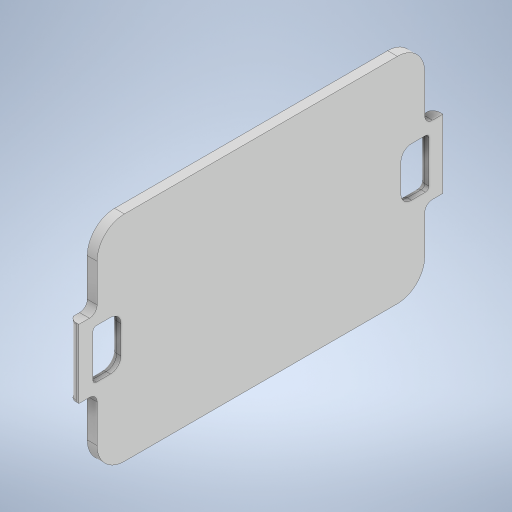
# Autodesk Inventor part: PlateGantryMountSpringRetainer
Saved by Autodesk Inventor 2023 (Build 270158000, 158)
## iProperties
Created: 2026-01-31
Part Number: PlateGantryMountSpringRetainer
Material: Generic
Document SubType Name: Modeling
Designer: DanAr
Density: 1 g/cm^3
Appearance: Default
Author: DanAr
Autodesk Inventor part; units mm, degrees
ref_plane "YZ Plane" through (0, 0, 0) normal (1, 0, 0) x (0, 1, 0)
ref_plane "XZ Plane" through (0, 0, 0) normal (0, 1, 0) x (-1, 0, 0)
ref_plane "XY Plane" through (0, 0, 0) normal (0, 0, 1) x (1, 0, 0)
sketch "Sketch1" plane through (0, 0, 0) normal (1, 0, 0) x (0, 1, 0)
  line L0 (-15.3, 23.4) -> (15.3, 23.4)
  line L1 (15.3, 23.4) -> (15.3, -23.4)
  line L2 (15.3, -23.4) -> (-15.3, -23.4)
  line L3 (-15.3, -23.4) -> (-15.3, 23.4)
  line L4 (-15.3, 23.4) -> (15.3, -23.4) construction
  line L5 (15.3, 23.4) -> (-15.3, -23.4) construction
  line L6 (-4.9, -26) -> (4.9, -26)
  line L7 (4.9, -26) -> (4.9, 26)
  line L8 (4.9, 26) -> (-4.9, 26)
  line L9 (-4.9, 26) -> (-4.9, -26)
  line L10 (-4.9, -26) -> (4.9, 26) construction
  line L11 (4.9, -26) -> (-4.9, 26) construction
  point P0 (0, 0)
  point P1 (-4.9, -23.4)
  point P2 (4.9, -23.4)
  point P3 (4.9, 23.4)
  point P4 (-4.9, 23.4)
  dimension "d0" = 46.8
  dimension "d1" = 30.6
  dimension "d2" = 52
  dimension "d3" = 9.8
  constraints: 24 end point, 4 midpoint, 4 parallel, 2 horizontal, 2 perpendicular
  measures "d0" distance of L0.end L1.end
  measures "d1" distance of L0.start L0.end
  measures "d2" distance of L6.end L7.end
  measures "d3" distance of L7.end L8.end
extrude "Extrusion1" add sketch "Sketch1" along normal blind 1.4
fillet "Fillet1" radius 1.1 4 edges at (0.7, 4.9, 23.4) (0.7, -4.9, 23.4) (0.7, 4.9, -23.4) (0.7, -4.9, -23.4)
fillet "Fillet2" radius 3.9 4 edges at (0.7, 15.3, 23.4) (0.7, 15.3, -23.4) (0.7, -15.3, 23.4) (0.7, -15.3, -23.4)
sketch "Sketch2" plane through (1.4, 0, 0) normal (1, 0, 0) x (0, 0, -1)
  line L0 (-26, 4.9) -> (-26, -4.9) projected
  line L1 (-26, 0) -> (-24, 0)
  line L2 (-24, 0) -> (-22, 0)
  line L3 (-20, -3.5) -> (-24, -3.5)
  line L4 (-24, -3.5) -> (-24, 3.5)
  line L5 (-24, 3.5) -> (-20, 3.5)
  line L6 (-20, 3.5) -> (-20, -3.5)
  line L7 (-20, -3.5) -> (-24, 3.5) construction
  line L8 (-24, -3.5) -> (-20, 3.5) construction
  line L9 (26, -4.9) -> (26, 4.9) projected
  line L10 (26, 0) -> (24, 0)
  line L11 (24, 0) -> (22, 0)
  line L12 (20, -3.5) -> (24, -3.5)
  line L13 (24, -3.5) -> (24, 3.5)
  line L14 (24, 3.5) -> (20, 3.5)
  line L15 (20, 3.5) -> (20, -3.5)
  line L16 (20, -3.5) -> (24, 3.5) construction
  line L17 (24, -3.5) -> (20, 3.5) construction
  point P0 (0, 0)
  dimension "d8" = 2
  dimension "d9" = 2
  dimension "d10" = 4
  dimension "d11" = 7
  dimension "d12" = 2
  dimension "d13" = 2
  dimension "d14" = 4
  dimension "d15" = 7
  constraints: 32 end point, 6 midpoint, 5 horizontal, 4 parallel, 2 perpendicular, 1 point on line
  measures "d8" distance of L1.start L1.end
  measures "d9" distance of L1.end L2.end
  measures "d10" distance of L4.end L5.end
  measures "d11" distance of L3.end L4.end
  measures "d12" distance of L10.start L10.end
  measures "d13" distance of L10.end L11.end
  measures "d14" distance of L13.end L14.end
  measures "d15" distance of L12.end L13.end
extrude "Extrusion2" cut sketch "Sketch2" against normal blind 1.4
fillet "Fillet3" radius 0.5 4 edges at (0.7, -3.5, -24) (0.7, 3.5, -24) (0.7, 3.5, 24) (0.7, -3.5, 24)
fillet "Fillet4" radius 1.5 4 edges at (0.7, -3.5, 20) (0.7, 3.5, 20) (0.7, 3.5, -20) (0.7, -3.5, -20)
fillet "Fillet5" radius 0.8 16 edges at (0, 0, 20) (0, 3.0607, 20.4393) (0, 3.5, 22.5) (0, 3.3536, 23.8536) (0, 0, 24) (0, -3.3536, 23.8536) (0, -3.5, 22.5) (0, -3.0607, 20.4393) (0, 3.3536, -23.8536) (0, 3.5, -22.5) (0, 3.0607, -20.4393) (0, 0, -20) (0, -3.0607, -20.4393) (0, -3.5, -22.5) (0, -3.3536, -23.8536) (0, 0, -24)
sketch "Sketch3" plane through (0, -4.9, 26) normal (0, 0, 1) x (1, 0, 0)
  line L0 (9.5754, -0.1) -> (-9.5754, -0.1)
  line L1 (-9.5754, -0.1) -> (-9.5754, 9.9)
  line L2 (-9.5754, 9.9) -> (9.5754, 9.9)
  line L3 (9.5754, 9.9) -> (9.5754, -0.1)
  line L4 (9.5754, -0.1) -> (-9.5754, 9.9) construction
  line L5 (-9.5754, -0.1) -> (9.5754, 9.9) construction
  line L6 (0, 10.9) -> (1.4, 10.9) projected
  line L7 (-19.1508, -1.1) -> (0, -1.1)
  line L8 (0, -1.1) -> (0, 10.9)
  line L9 (0, 10.9) -> (-19.1508, 10.9)
  line L10 (-19.1508, 10.9) -> (-19.1508, -1.1)
  line L11 (-19.1508, -1.1) -> (0, 10.9) construction
  line L12 (0, -1.1) -> (-19.1508, 10.9) construction
  line L13 (0, -1.1) -> (1.4, -1.1) projected
  line L14 (0, 10.9) -> (1.4, 10.9)
  line L15 (1.4, 10.9) -> (1.4, -1.1)
  line L16 (1.4, -1.1) -> (0, -1.1)
  line L17 (0, -1.1) -> (0, 10.9)
  line L18 (1.4, 9.8) -> (0, 9.8) projected
  line L19 (1.4, 0) -> (1.4, 9.8) projected
  line L20 (0, 9.8) -> (1.4, 9.8)
  line L21 (1.4, 9.8) -> (1.4, 0)
  line L22 (1.4, 0) -> (0, 0)
  line L23 (0, 0) -> (0, 9.8)
  line L24 (0, -3.3408) -> (-19.1508, -3.3408)
  line L25 (-19.1508, -3.3408) -> (-19.1508, 13.1408)
  line L26 (-19.1508, 13.1408) -> (0, 13.1408)
  line L27 (0, 13.1408) -> (0, -3.3408)
  line L28 (0, -3.3408) -> (-19.1508, 13.1408) construction
  line L29 (-19.1508, -3.3408) -> (0, 13.1408) construction
  line L30 (1.4, -6.5) -> (1.4, -1.1) projected
  line L31 (0, 13.1408) -> (1.4, 13.1408)
  line L32 (1.4, 13.1408) -> (1.4, -3.3408)
  line L33 (1.4, -3.3408) -> (0, -3.3408)
  line L34 (0, -3.3408) -> (0, 13.1408)
  point P0 (0, 4.9)
  point P1 (-9.5754, 4.9)
  point P2 (0, -0.1)
  point P3 (0, 9.9)
  point P4 (0, -3.3408)
  dimension "d21" = 10
  dimension "d29" = 12
  constraints: 60 end point, 12 parallel, 7 midpoint, 6 horizontal, 6 perpendicular, 1 point on line
  measures "d21" distance of L0.end L1.end
  measures "d29" distance of L9.end L7.start
extrude "Extrusion3" add sketch "Sketch3" against normal blind 2.5 contours L15 L13 L8 L0 | L0 L8 L22 L15 | L8 L7 L10 L9 L2 L1 L0 | L30 L33 L27 L13 | L15 L18 L8 L2 | L2 L8 L6 L15 | L27 L24 L25 L7 | L6 L27 L31 L32 | L9 L25 L26 L27
sketch "Sketch4" plane through (0, -4.9, -26) normal (0, 0, -1) x (-1, 0, 0)
  line L0 (9.5754, 9.9) -> (0, 9.9) projected
  line L1 (0, -0.1) -> (9.5754, -0.1) projected
  line L2 (9.5754, 9.9) -> (0, 9.9)
  line L3 (0, 9.9) -> (0, -0.1)
  line L4 (0, -0.1) -> (9.5754, -0.1)
  line L5 (9.5754, -0.1) -> (9.5754, 9.9)
  line L6 (0, 0) -> (-1.4, 0) projected
  line L7 (0, -0.1) -> (-1.4, -0.1)
  line L8 (-1.4, -0.1) -> (-1.4, 0)
  line L9 (-1.4, 0) -> (0, 0)
  line L10 (0, 0) -> (0, -0.1)
  line L11 (-1.4, -0.1) -> (9.5754, -0.1)
  line L12 (9.5754, -0.1) -> (9.5754, -1.1)
  line L13 (9.5754, -1.1) -> (-1.4, -1.1)
  line L14 (-1.4, -1.1) -> (-1.4, -0.1)
  line L15 (0, 9.9) -> (0, -0.1) projected
  line L16 (-1.4, 9.8) -> (0, 9.8) projected
  line L17 (0, 9.9) -> (-1.4, 9.9)
  line L18 (-1.4, 9.9) -> (-1.4, 9.8)
  line L19 (-1.4, 9.8) -> (0, 9.8)
  line L20 (0, 9.8) -> (0, 9.9)
  line L21 (-1.4, 10.9) -> (19.1508, 10.9) projected
  line L22 (-1.4, 9.9) -> (9.5754, 9.9)
  line L23 (9.5754, 9.9) -> (9.5754, 10.9)
  line L24 (9.5754, 10.9) -> (-1.4, 10.9)
  line L25 (-1.4, 10.9) -> (-1.4, 9.9)
  line L26 (19.1508, 10.9) -> (-1.4, 10.9) projected
  line L27 (-1.4, 10.9) -> (9.5754, 10.9)
  line L28 (9.5754, 10.9) -> (9.5754, 11.6514)
  line L29 (9.5754, 11.6514) -> (-1.4, 11.6514)
  line L30 (-1.4, 11.6514) -> (-1.4, 10.9)
  line L31 (-1.4, -1.1) -> (0, -1.1) projected
  line L32 (-1.4, -1.1) -> (9.5754, -1.1)
  line L33 (9.5754, -1.1) -> (9.5754, -1.8821)
  line L34 (9.5754, -1.8821) -> (-1.4, -1.8821)
  line L35 (-1.4, -1.8821) -> (-1.4, -1.1)
  point P0 (0, 4.9)
  constraints: 56 end point, 14 parallel, 7 horizontal, 7 perpendicular, 4 point on line
extrude "Extrusion4" add sketch "Sketch4" against normal blind 2.5 contours L0 L17 L25 L21 L23 | L3 L16 L18 L17 | L12 L13 L14 L7 L1 | L21 L30 L29 L28 | L7 L8 L6 L3 | L33 L34 L35 L13
fillet "Fillet7" radius 0.3 4 edges at (0, -5, -24.75) (0, 5, -24.75) (0, -5, 24.75) (0, 5, 24.75)
fillet "Fillet8" radius 1 9 edges at (-4.9377, -5, -26) (-0.0879, -4.9121, -26) (0, 0, -26) (-0.0879, 4.9121, -26) (-4.9377, 5, -26) (-0.0879, -4.9121, -23.5) (-4.9377, -5, -23.5) (-0.0879, 4.9121, -23.5) (-4.9377, 5, -23.5)
fillet "Fillet9" radius 1 9 edges at (-4.9377, -5, 23.5) (-0.0879, -4.9121, 23.5) (-0.0879, -4.9121, 26) (0, 0, 26) (-0.0879, 4.9121, 26) (-4.9377, 5, 26) (-4.9377, -5, 26) (-0.0879, 4.9121, 23.5) (-4.9377, 5, 23.5)
sketch "Sketch5" plane through (0, 0, 0) normal (-1, 0, 0) x (0, 0, 1)
  arc A0 (-23.5, 5.5417) -> (-23.4, 6) centre (-24.5, 6) ccw projected
  circle A1 centre (-24.5, 6) radius 1.1
  line L0 (-26, 6.7514) -> (-23.5, 6.7514) projected
  arc A2 (-24.5, 5) -> (-23.5, 6) centre (-24.5, 6) ccw projected
  line L1 (-26, 6.7514) -> (-23.5, 6.7514)
  line L2 (-23.5, 6.7514) -> (-23.5, 6)
  line L3 (-23.5, 6) -> (-26, 6)
  line L4 (-26, 6) -> (-26, 6.7514)
  line L5 (-24.5, 5) -> (-24.5, 4.7) projected
  line L6 (-26, 6.7514) -> (-26, -6.7821) projected
  line L7 (-24.5, 4.9) -> (-26, 4.9)
  line L8 (-26, 4.9) -> (-26, 6.7514)
  line L9 (-26, 6.7514) -> (-24.5, 6.7514)
  line L10 (-24.5, 6.7514) -> (-24.5, 4.9)
  arc A3 (-23.4, -6) -> (-23.977, -5.0323) centre (-24.5, -6) ccw projected
  circle A4 centre (-24.5, -6) radius 1.1
  line L11 (-24.5, -4.7) -> (-24.5, -5) projected
  line L12 (-24.5, -4.9) -> (-26, -4.9)
  line L13 (-26, -4.9) -> (-26, -6.7821)
  line L14 (-26, -6.7821) -> (-24.5, -6.7821)
  line L15 (-24.5, -6.7821) -> (-24.5, -4.9)
  line L16 (-23.5, -6.7821) -> (-26, -6.7821)
  line L17 (-26, -6.7821) -> (-26, -4.9)
  line L18 (-26, -4.9) -> (-23.5, -4.9)
  line L19 (-23.5, -4.9) -> (-23.5, -6.7821)
  point P0 (0, 0)
  point P1 (-23.5, 6.4583)
  point P2 (-23.6967, 6.7514)
  point P3 (-25.3033, 6.7514)
  constraints: 32 end point, 8 parallel, 4 horizontal, 4 perpendicular, 4 point on circle, 2 centre point, 2 coincident, 2 point on line
extrude "Extrusion5" cut sketch "Sketch5" along normal blind 20 contours A1 L5 A2 L2 A0 | L7 L6 L3 A1 | A1 L3 L10 L5 | L2 L3 L10 L0 A1 | A1 L0 L2 | L3 L4 L0 A1 | A1 L0 L10 L3 | L10 L3 A2 | L0 A1
sketch "Sketch6" plane through (-19.1508, 8.2408, 26) normal (0, 0, 1) x (1, 0, 0)
  line L0 (20.5508, 0) -> (0, 0) projected
  line L1 (0, -16.4817) -> (20.5508, -16.4817) projected
  line L2 (0, 0) -> (19.1508, 0)
  line L3 (19.1508, 0) -> (19.1508, -16.4817)
  line L4 (19.1508, -16.4817) -> (0, -16.4817)
  line L5 (0, -16.4817) -> (0, 0)
  point P0 (19.1508, -8.2408)
  constraints: 8 end point, 2 parallel, 1 horizontal, 1 perpendicular, 1 point on line
extrude "Extrusion6" cut sketch "Sketch6" against normal blind 200
sketch "Sketch7" plane through (0, 0, 0) normal (-1, 0, 0) x (0, 0, 1)
  arc A0 (-23.977, 5.0323) -> (-23.4, 6) centre (-24.5, 6) ccw projected
  circle A1 centre (-24.5, 6) radius 1.1
  arc A2 (-23.4, -6) -> (-23.977, -5.0323) centre (-24.5, -6) ccw projected
  line L0 (-23.4, -11.4) -> (-23.4, -6) projected
  circle A3 centre (-24.5, -6) radius 1.1
  arc A4 (23.977, -5.0323) -> (23.4, -6) centre (24.5, -6) ccw projected
  circle A5 centre (24.5, -6) radius 1.1
  arc A6 (23.4, 6) -> (23.977, 5.0323) centre (24.5, 6) ccw projected
  circle A7 centre (24.5, 6) radius 1.1
  line L1 (23.5, 5.9649) -> (23.5, 8.2408) projected
  line L2 (26, 4.7) -> (26, 5.9649) projected
  line L3 (23.5, 8.2408) -> (26, 8.2408)
  line L4 (26, 8.2408) -> (26, 4.9)
  line L5 (26, 4.9) -> (23.5, 4.9)
  line L6 (23.5, 4.9) -> (23.5, 8.2408)
  line L7 (26, -8.2408) -> (23.5, -8.2408) projected
  line L8 (26, -8.2408) -> (23.4, -8.2408)
  line L9 (23.4, -8.2408) -> (23.4, -4.9)
  line L10 (23.4, -4.9) -> (26, -4.9)
  line L11 (26, -4.9) -> (26, -8.2408)
  line L12 (-26, -6.7821) -> (-26, -5.9649) projected
  line L13 (-26, -6.7821) -> (-24.5, -6.7821)
  line L14 (-24.5, -6.7821) -> (-24.5, -4.9)
  line L15 (-24.5, -4.9) -> (-26, -4.9)
  line L16 (-26, -4.9) -> (-26, -6.7821)
  line L17 (-23.5, -5.9649) -> (-23.5, -6.7821) projected
  line L18 (-23.5, -6.7821) -> (-24.5, -6.7821)
  line L19 (-24.5, -6.7821) -> (-24.5, -6)
  line L20 (-24.5, -6) -> (-23.5, -6)
  line L21 (-23.5, -6) -> (-23.5, -6.7821)
  line L22 (-26, 6.7514) -> (-23.5, 6.7514) projected
  line L23 (-26, 6.7514) -> (-23.5, 6.7514)
  line L24 (-23.5, 6.7514) -> (-23.5, 4.9)
  line L25 (-23.5, 4.9) -> (-26, 4.9)
  line L26 (-26, 4.9) -> (-26, 6.7514)
  point P0 (0, 0)
  point P1 (23.5, 5.5417)
  point P2 (23.977, 5.0323)
  point P3 (24.5, 4.9)
  point P4 (24.5, -4.9)
  point P5 (-25.2735, -6.7821)
  point P6 (-23.7265, -6.7821)
  point P7 (-23.5, -6.4583)
  point P8 (-23.977, -5.0323)
  point P9 (-24.5, 4.9)
  point P10 (-23.977, 5.0323)
  point P11 (-23.5, 6.4583)
  point P12 (-23.6967, 6.7514)
  point P13 (-25.3033, 6.7514)
  constraints: 40 end point, 10 parallel, 5 horizontal, 5 perpendicular, 4 coincident, 4 point on line, 2 point on circle, 1 centre point, 9 other
extrude "Extrusion7" cut sketch "Sketch7" against normal blind 20 contours A1 L22 L24 A0 | L24 A1 A0 | L25 L26 L22 A1 | A1 L22 L24 | A1 L22 | A3 L17 L20 L14 A2 | L17 L18 A3 | A3 L18 L14 L20 L17 | L14 L13 A3 | A3 L13 L12 L16 L15 | A3 L13 L18 | A5 A4 | A5 L10 L11 L7 L8 L9 | L6 L1 A7 A6 | L1 L3 L4 L2 L5 A7 picked at (24.8889, 6.0778)
body "Solid1"
